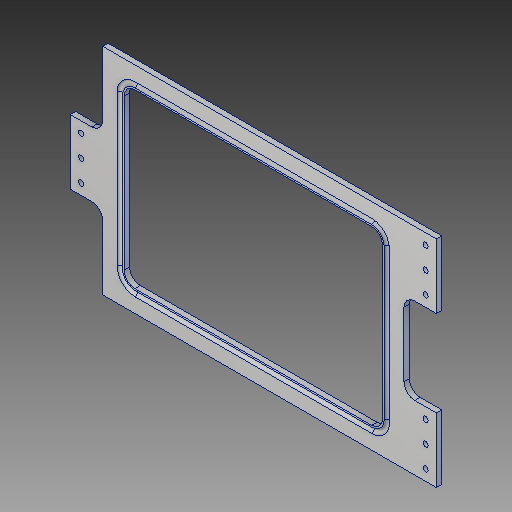
# Autodesk Inventor part: top
Saved by Autodesk Inventor 2018.1 (Build 221171000, 171)
## iProperties
Created: 2017-07-28
Part Number: top
Material: Aluminum 6061
Document SubType Name: Modeling
Designer: Kai
Density: 2.7 g/cm^3
Appearance: Aluminum - Flat
Author: Kai
Autodesk Inventor part; units mm, degrees
ref_plane "YZ Plane" through (0, 0, 0) normal (1, 0, 0) x (0, 1, 0)
ref_plane "XZ Plane" through (0, 0, 0) normal (0, 1, 0) x (-1, 0, 0)
sketch "Sketch1" plane through (0, 0, 0) normal (0, 0, 1) x (1, 0, 0)
  line L0 (0, 0) -> (-355.6, 0)
  line L1 (-355.6, 0) -> (-355.6, 254)
  line L2 (-355.6, 254) -> (0, 254)
  line L3 (0, 254) -> (0, 0)
  line L4 (-38.1, 25.4) -> (-317.5, 25.4)
  line L5 (-330.2, 38.1) -> (-330.2, 215.9)
  line L6 (-317.5, 228.6) -> (-38.1, 228.6)
  line L7 (-25.4, 215.9) -> (-25.4, 38.1)
  line L8 (-12.7, 241.3) -> (-342.9, 241.3) construction
  line L9 (-342.9, 241.3) -> (-342.9, 12.7) construction
  line L10 (-342.9, 12.7) -> (-12.7, 12.7) construction
  line L11 (-12.7, 12.7) -> (-12.7, 241.3) construction
  circle A0 centre (-342.9, 241.3) radius 3.1
  circle A1 centre (-342.9, 215.9) radius 3.1
  circle A2 centre (-342.9, 190.5) radius 3.1
  circle A3 centre (-342.9, 165.1) radius 3.1
  circle A4 centre (-342.9, 139.7) radius 3.1
  circle A5 centre (-342.9, 114.3) radius 3.1
  circle A6 centre (-342.9, 88.9) radius 3.1
  circle A7 centre (-342.9, 63.5) radius 3.1
  circle A8 centre (-342.9, 38.1) radius 3.1
  circle A9 centre (-342.9, 12.7) radius 3.1
  circle A10 centre (-317.5, 241.3) radius 3.1
  circle A11 centre (-292.1, 241.3) radius 3.1
  circle A12 centre (-266.7, 241.3) radius 3.1
  circle A13 centre (-241.3, 241.3) radius 3.1
  circle A14 centre (-215.9, 241.3) radius 3.1
  circle A15 centre (-190.5, 241.3) radius 3.1
  circle A16 centre (-165.1, 241.3) radius 3.1
  circle A17 centre (-139.7, 241.3) radius 3.1
  circle A18 centre (-114.3, 241.3) radius 3.1
  circle A19 centre (-88.9, 241.3) radius 3.1
  circle A20 centre (-63.5, 241.3) radius 3.1
  circle A21 centre (-38.1, 241.3) radius 3.1
  circle A22 centre (-12.7, 241.3) radius 3.1
  circle A23 centre (-12.7, 215.9) radius 3.1
  circle A24 centre (-12.7, 190.5) radius 3.1
  circle A25 centre (-12.7, 165.1) radius 3.1
  circle A26 centre (-12.7, 139.7) radius 3.1
  circle A27 centre (-12.7, 114.3) radius 3.1
  circle A28 centre (-12.7, 88.9) radius 3.1
  circle A29 centre (-12.7, 63.5) radius 3.1
  circle A30 centre (-12.7, 38.1) radius 3.1
  circle A31 centre (-12.7, 12.7) radius 3.1
  circle A32 centre (-38.1, 12.7) radius 3.1
  circle A33 centre (-63.5, 12.7) radius 3.1
  circle A34 centre (-88.9, 12.7) radius 3.1
  circle A35 centre (-114.3, 12.7) radius 3.1
  circle A36 centre (-139.7, 12.7) radius 3.1
  circle A37 centre (-165.1, 12.7) radius 3.1
  circle A38 centre (-190.5, 12.7) radius 3.1
  circle A39 centre (-215.9, 12.7) radius 3.1
  circle A40 centre (-241.3, 12.7) radius 3.1
  circle A41 centre (-266.7, 12.7) radius 3.1
  circle A42 centre (-292.1, 12.7) radius 3.1
  circle A43 centre (-317.5, 12.7) radius 3.1
  arc A44 (-317.5, 228.6) -> (-330.2, 215.9) centre (-317.5, 215.9) ccw
  arc A45 (-330.2, 38.1) -> (-317.5, 25.4) centre (-317.5, 38.1) ccw
  arc A46 (-38.1, 25.4) -> (-25.4, 38.1) centre (-38.1, 38.1) ccw
  arc A47 (-25.4, 215.9) -> (-38.1, 228.6) centre (-38.1, 215.9) ccw
  dimension "d0" = 355.6
  dimension "d1" = 254
  dimension "d2" = 25.4
  dimension "d3" = 12.7
  dimension "d4" = 6.2
  dimension "d7" = 25.4
  dimension "d14" = 25.4
  dimension "d21" = 25.4
  dimension "d28" = 25.4
  dimension "d33" = 12.7
  constraints: 48 centre point, 24 end point, 8 point on circle, 8 tangent, 6 parallel, 3 equal radius, 3 horizontal, 3 perpendicular, 2 vertical, 1 coincident, 92 other
  measures "d0" distance of L1.end L2.end
  measures "d1" distance of L0.end L1.end
  measures "d2" distance between parallel lines of L3 L7
  measures "d3" distance between parallel lines of L2 L8
  measures "d4" diameter of A0
  measures "d7" distance of A0.centre A1.centre
  measures "d14" distance of A0.centre A10.centre
  measures "d21" distance of A22.centre A23.centre
  measures "d28" distance of A31.centre A32.centre
  measures "d33" radius of A44
extrude "Extrusion1" add sketch "Sketch1" along normal blind 6.35
sketch "Sketch5" plane through (0, 0, 6.35) normal (0, 0, 1) x (1, 0, 0)
  arc A0 (-38.1, 25.4) -> (-25.4, 38.1) centre (-38.1, 38.1) ccw construction
  circle A1 centre (-12.7, 38.1) radius 3.1 construction
  circle A2 centre (-38.1, 38.1) radius 25.4 construction
  arc A3 (-330.2, 38.1) -> (-317.5, 25.4) centre (-317.5, 38.1) ccw construction
  circle A4 centre (-317.5, 38.1) radius 25.4 construction
  circle A5 centre (-342.9, 215.9) radius 3.1 construction
  circle A6 centre (-317.5, 215.9) radius 25.4 construction
  circle A7 centre (-12.7, 215.9) radius 3.1 construction
  circle A8 centre (-38.1, 215.9) radius 25.4 construction
  line L0 (-38.1, 215.9) -> (-20.1395, 233.8605) construction
  line L1 (-38.1, 215.9) -> (-12.7, 215.9) construction
  line L2 (-38.1, 38.1) -> (-20.1395, 20.1395) construction
  line L3 (-317.5, 38.1) -> (-335.4605, 20.1395) construction
  line L4 (-317.5, 215.9) -> (-335.4605, 233.8605) construction
  circle A9 centre (-335.4605, 233.8605) radius 3.1
  circle A10 centre (-20.1395, 233.8605) radius 3.1
  circle A11 centre (-20.1395, 20.1395) radius 3.1
  circle A12 centre (-335.4605, 20.1395) radius 3.1
  point P0 (0, 0)
  dimension "d49" = 45
  dimension "d50" = 6.2
  dimension "d51" = 6.2
  dimension "d52" = 6.2
  dimension "d53" = 6.2
  constraints: 10 end point, 7 centre point, 6 coincident, 6 point on circle, 2 perpendicular, 1 equal length, 1 horizontal, 3 other
  measures "d49" angle of L1 L0
  measures "d50" diameter of A9
  measures "d51" diameter of A10
  measures "d52" diameter of A11
  measures "d53" diameter of A12
extrude "Extrusion3" cut sketch "Sketch5" against normal blind 6.35
sketch "Sketch9" plane through (0, 0, 6.35) normal (0, 0, 1) x (1, 0, 0)
  circle A0 centre (-20.1395, 20.1395) radius 3.1 projected
  circle A1 centre (-20.1395, 20.1395) radius 3.1
  circle A2 centre (-38.1, 12.7) radius 3.1 projected
  circle A3 centre (-38.1, 12.7) radius 3.1
  circle A4 centre (-335.4605, 20.1395) radius 3.1 projected
  circle A5 centre (-335.4605, 20.1395) radius 3.1
  circle A6 centre (-335.4605, 233.8605) radius 3.1 projected
  circle A7 centre (-335.4605, 233.8605) radius 3.1
  circle A8 centre (-20.1395, 233.8605) radius 3.1 projected
  circle A9 centre (-20.1395, 233.8605) radius 3.1
  circle A10 centre (-38.1, 241.3) radius 3.1 projected
  circle A11 centre (-38.1, 241.3) radius 3.1
  circle A12 centre (-266.7, 241.3) radius 3.1 projected
  line L0 (-266.7, 241.3) -> (-275.1476, 241.3) construction
  line L1 (-292.1, 241.3) -> (-300.5476, 241.3) construction
  circle A13 centre (-63.5, 241.3) radius 3.1
  line L2 (-317.5, 241.3) -> (-325.9476, 241.3) construction
  circle A14 centre (-88.9, 241.3) radius 3.1
  line L3 (-342.9, 241.3) -> (-351.3476, 241.3) construction
  circle A15 centre (-114.3, 241.3) radius 3.1
  line L4 (-368.3, 241.3) -> (-376.7476, 241.3) construction
  circle A16 centre (-139.7, 241.3) radius 3.1
  line L5 (-393.7, 241.3) -> (-402.1476, 241.3) construction
  circle A17 centre (-165.1, 241.3) radius 3.1
  line L6 (-419.1, 241.3) -> (-427.5476, 241.3) construction
  circle A18 centre (-190.5, 241.3) radius 3.1
  line L7 (-444.5, 241.3) -> (-452.9476, 241.3) construction
  circle A19 centre (-215.9, 241.3) radius 3.1
  line L8 (-469.9, 241.3) -> (-478.3476, 241.3) construction
  circle A20 centre (-241.3, 241.3) radius 3.1
  line L9 (-495.3, 241.3) -> (-503.7476, 241.3) construction
  circle A21 centre (-266.7, 241.3) radius 3.1
  line L10 (-520.7, 241.3) -> (-529.1476, 241.3) construction
  circle A22 centre (-292.1, 241.3) radius 3.1
  line L11 (-546.1, 241.3) -> (-554.5476, 241.3) construction
  circle A23 centre (-317.5, 241.3) radius 3.1
  circle A24 centre (-342.9, 215.9) radius 3.1 projected
  circle A25 centre (-342.9, 215.9) radius 3.1
  line L12 (-342.9, 190.5569) -> (-342.9, 174.56) construction
  circle A26 centre (-63.5, 12.7) radius 3.1 construction
  line L13 (-63.5, 12.7) -> (-88.9, 12.7) construction
  circle A27 centre (-12.7, 38.1) radius 3.1 construction
  circle A28 centre (-12.7, 63.5) radius 3.1 construction
  line L14 (-12.7, 38.1) -> (-12.7, 63.5) construction
  circle A29 centre (-12.7, 215.9) radius 3.1 projected
  circle A30 centre (-12.7, 215.9) radius 3.1
  circle A31 centre (-12.7, 190.5) radius 3.1
  circle A32 centre (-12.7, 165.1) radius 3.1
  circle A33 centre (-12.7, 139.7) radius 3.1
  circle A34 centre (-12.7, 114.3) radius 3.1
  circle A35 centre (-12.7, 88.9) radius 3.1
  circle A36 centre (-12.7, 63.5) radius 3.1
  circle A37 centre (-12.7, 38.1) radius 3.1
  circle A38 centre (-63.5, 12.7) radius 3.1
  circle A39 centre (-88.9, 12.7) radius 3.1
  circle A40 centre (-114.3, 12.7) radius 3.1
  circle A41 centre (-139.7, 12.7) radius 3.1
  circle A42 centre (-165.1, 12.7) radius 3.1
  circle A43 centre (-190.5, 12.7) radius 3.1
  circle A44 centre (-215.9, 12.7) radius 3.1
  circle A45 centre (-241.3, 12.7) radius 3.1
  circle A46 centre (-266.7, 12.7) radius 3.1
  circle A47 centre (-292.1, 12.7) radius 3.1
  circle A48 centre (-317.5, 12.7) radius 3.1
  circle A49 centre (-342.9, 190.5) radius 3.1
  circle A50 centre (-342.9, 165.1) radius 3.1
  circle A51 centre (-342.9, 139.7) radius 3.1
  circle A52 centre (-342.9, 114.3) radius 3.1
  circle A53 centre (-342.9, 88.9) radius 3.1
  circle A54 centre (-342.9, 63.5) radius 3.1
  circle A55 centre (-342.9, 38.1) radius 3.1
  line L15 (-355.6, 254) -> (0, 254) projected
  line L16 (-355.6, 254) -> (0, 254)
  line L17 (0, 254) -> (0, 0)
  line L18 (0, 0) -> (-355.6, 0)
  line L19 (-355.6, 0) -> (-355.6, 254)
  dimension "d66" = 25.4
  dimension "d73" = 25.4
  dimension "d80" = 25.4
  dimension "d87" = 25.4
  constraints: 44 centre point, 38 end point, 8 coincident, 5 horizontal, 4 vertical, 2 parallel, 1 collinear, 1 perpendicular, 104 other
  measures "d66" distance of L0.start L1.start
  measures "d73" distance of A30.centre A31.centre
  measures "d80" distance of A3.centre A38.centre
  measures "d87" distance of A25.centre A49.centre
extrude "Extrusion4" add sketch "Sketch9" against normal blind 12.7
sketch "Sketch10" plane through (0, 0, 6.35) normal (0, 0, 1) x (1, 0, 0)
  line L0 (-355.6, 0) -> (-355.6, 254) construction
  line L1 (0, 0) -> (-355.6, 0) construction
  line L2 (-355.6, 0) -> (-355.6, 254) construction
  line L3 (-355.6, 254) -> (0, 254) construction
  line L4 (0, 254) -> (0, 0) construction
  line L5 (-38.1, 228.6) -> (-317.5, 228.6)
  line L6 (-330.2, 215.9) -> (-330.2, 38.1)
  line L7 (-317.5, 25.4) -> (-38.1, 25.4)
  line L8 (-25.4, 38.1) -> (-25.4, 215.9)
  arc A0 (-317.5, 228.6) -> (-330.2, 215.9) centre (-317.5, 215.9) ccw
  arc A1 (-25.4, 215.9) -> (-38.1, 228.6) centre (-38.1, 215.9) ccw
  arc A2 (-38.1, 25.4) -> (-25.4, 38.1) centre (-38.1, 38.1) ccw
  arc A3 (-330.2, 38.1) -> (-317.5, 25.4) centre (-317.5, 38.1) ccw
  dimension "d94" = 25.4
  dimension "d95" = 12.7
  constraints: 16 end point, 8 point on circle, 8 tangent, 4 centre point, 4 parallel, 3 equal radius, 2 perpendicular, 1 horizontal, 3 other
  measures "d94" distance between parallel lines of L3 L5
  measures "d95" radius of A0
extrude "Extrusion5" cut sketch "Sketch10" against normal blind 25.4
sketch "Sketch11" plane through (0, 0, -6.35) normal (0, 0, -1) x (-1, 0, 0)
  line L0 (355.6, 0) -> (355.6, 254) projected
  line L1 (0, 0) -> (355.6, 0)
  line L2 (355.6, 0) -> (355.6, 254)
  line L3 (355.6, 254) -> (0, 254)
  line L4 (0, 254) -> (0, 0)
  constraints: 8 end point, 2 parallel, 1 horizontal, 1 perpendicular
extrude "Extrusion6" cut sketch "Sketch11" against normal blind 6.35
sketch "Sketch12" plane through (0, 0, 6.35) normal (0, 0, 1) x (1, 0, 0)
  line L0 (-38.1, 20.32) -> (-317.5, 20.32)
  line L1 (-335.28, 38.1) -> (-335.28, 215.9)
  line L2 (-317.5, 233.68) -> (-38.1, 233.68)
  line L3 (-20.32, 215.9) -> (-20.32, 38.1)
  line L4 (-355.6, 254) -> (-355.6, 0) projected
  line L5 (-355.6, 0) -> (0, 0) projected
  arc A0 (-335.28, 38.1) -> (-317.5, 20.32) centre (-317.5, 38.1) ccw
  arc A1 (-317.5, 233.68) -> (-335.28, 215.9) centre (-317.5, 215.9) ccw
  arc A2 (-20.32, 215.9) -> (-38.1, 233.68) centre (-38.1, 215.9) ccw
  arc A3 (-38.1, 20.32) -> (-20.32, 38.1) centre (-38.1, 38.1) ccw
  point P0 (-335.28, 233.68)
  point P1 (-335.28, 20.32)
  point P2 (-20.32, 233.68)
  dimension "d100" = 314.96
  dimension "d101" = 213.36
  dimension "d102" = 20.32
  dimension "d103" = 20.32
  dimension "d104" = 17.78
  constraints: 8 end point, 8 point on circle, 8 tangent, 6 point on line, 4 centre point, 3 equal radius, 2 parallel, 1 horizontal, 1 perpendicular
  measures "d100" distance of point (-335.28, 233.68) point (-20.32, 233.68)
  measures "d101" distance of point (-335.28, 20.32) point (-335.28, 233.68)
  measures "d102" distance between parallel lines of L4 L1
  measures "d103" distance between parallel lines of L5 L0
  measures "d104" radius of A0
ref_plane "Work Plane2" through (-279.4, 38.1, 6.35) normal (1, 0, 0) x (0, 0, -1)
sketch "Sketch13" plane through (-279.4, 38.1, 6.35) normal (1, 0, 0) x (0, 0, -1)
  line L0 (0, 215.9) -> (0, -38.1) projected
  circle A0 centre (0, -17.78) radius 3.175
  line L1 (0, -38.1) -> (6.35, -38.1) projected
  dimension "d106" = 6.35
  dimension "d107" = 20.32
  constraints: 1 centre point, 1 point on line
  measures "d106" diameter of A0
  measures "d107" distance from line of L1 A0.centre
sweep "Sweep3" cut profiles "Sketch13" path "Sketch12" path curves L0 A3 L3 A2 L2 A1 L1 A0
sketch "Sketch14" plane through (0, 0, 6.35) normal (0, 0, 1) x (1, 0, 0)
  circle A0 centre (-20.1395, 20.1395) radius 3.1 projected
  circle A1 centre (-20.1395, 20.1395) radius 3.1
  circle A2 centre (-38.1, 12.7) radius 3.1 projected
  circle A3 centre (-38.1, 12.7) radius 3.1
  circle A4 centre (-12.7, 38.1) radius 3.1 projected
  circle A5 centre (-12.7, 38.1) radius 3.1
  circle A6 centre (-20.1395, 233.8605) radius 3.1 projected
  circle A7 centre (-20.1395, 233.8605) radius 3.1
  circle A8 centre (-38.1, 241.3) radius 3.1 projected
  circle A9 centre (-38.1, 241.3) radius 3.1
  circle A10 centre (-335.4605, 233.8605) radius 3.1 projected
  circle A11 centre (-335.4605, 233.8605) radius 3.1
  circle A12 centre (-335.4605, 20.1395) radius 3.1 projected
  circle A13 centre (-335.4605, 20.1395) radius 3.1
  circle A14 centre (-342.9, 38.1) radius 3.1 projected
  circle A15 centre (-342.9, 38.1) radius 3.1
  circle A16 centre (-292.1, 12.7) radius 3.1 construction
  circle A17 centre (-266.7, 12.7) radius 3.1 construction
  line L0 (-292.1, 12.7) -> (-266.7, 12.7) construction
  circle A18 centre (-342.9, 63.5) radius 3.1 construction
  circle A19 centre (-342.9, 88.9) radius 3.1 construction
  line L1 (-342.9, 63.5) -> (-342.9, 88.9) construction
  circle A20 centre (-292.1, 241.3) radius 3.1 construction
  line L2 (-292.1, 241.3) -> (-266.7, 241.3) construction
  circle A21 centre (-12.7, 215.9) radius 3.1 construction
  circle A22 centre (-12.7, 190.5) radius 3.1 construction
  line L3 (-12.7, 215.9) -> (-12.7, 190.5) construction
  circle A23 centre (-63.5, 241.3) radius 3.1
  circle A24 centre (-88.9, 241.3) radius 3.1
  circle A25 centre (-114.3, 241.3) radius 3.1
  circle A26 centre (-139.7, 241.3) radius 3.1
  circle A27 centre (-165.1, 241.3) radius 3.1
  circle A28 centre (-190.5, 241.3) radius 3.1
  circle A29 centre (-215.9, 241.3) radius 3.1
  circle A30 centre (-241.3, 241.3) radius 3.1
  circle A31 centre (-266.7, 241.3) radius 3.1
  circle A32 centre (-292.1, 241.3) radius 3.1
  circle A33 centre (-317.5, 241.3) radius 3.1
  circle A34 centre (-12.7, 63.5) radius 3.1
  circle A35 centre (-12.7, 88.9) radius 3.1
  circle A36 centre (-12.7, 114.3) radius 3.1
  circle A37 centre (-12.7, 139.7) radius 3.1
  circle A38 centre (-12.7, 165.1) radius 3.1
  circle A39 centre (-12.7, 190.5) radius 3.1
  circle A40 centre (-12.7, 215.9) radius 3.1
  circle A41 centre (-63.5, 12.7) radius 3.1
  circle A42 centre (-88.9, 12.7) radius 3.1
  circle A43 centre (-114.3, 12.7) radius 3.1
  circle A44 centre (-139.7, 12.7) radius 3.1
  circle A45 centre (-165.1, 12.7) radius 3.1
  circle A46 centre (-190.5, 12.7) radius 3.1
  circle A47 centre (-215.9, 12.7) radius 3.1
  circle A48 centre (-241.3, 12.7) radius 3.1
  circle A49 centre (-266.7, 12.7) radius 3.1
  circle A50 centre (-292.1, 12.7) radius 3.1
  circle A51 centre (-317.5, 12.7) radius 3.1
  circle A52 centre (-342.9, 63.5) radius 3.1
  circle A53 centre (-342.9, 88.9) radius 3.1
  circle A54 centre (-342.9, 114.3) radius 3.1
  circle A55 centre (-342.9, 139.7) radius 3.1
  circle A56 centre (-342.9, 165.1) radius 3.1
  circle A57 centre (-342.9, 190.5) radius 3.1
  circle A58 centre (-342.9, 215.9) radius 3.1
  point P0 (0, 0)
  dimension "d112" = 25.4
  dimension "d119" = 25.4
  dimension "d126" = 25.4
  dimension "d133" = 25.4
  constraints: 44 centre point, 8 coincident, 8 end point, 4 horizontal, 4 vertical, 72 other
  measures "d112" distance of A9.centre A23.centre
  measures "d119" distance of A5.centre A34.centre
  measures "d126" distance of A3.centre A41.centre
  measures "d133" distance of A15.centre A52.centre
extrude "Extrusion7" add sketch "Sketch14" against normal blind 6.35
sketch "Sketch15" plane through (0, 0, 6.35) normal (0, 0, 1) x (1, 0, 0)
  line L0 (-355.6, 254) -> (-355.6, 0) projected
  line L1 (-355.6, 165.1) -> (-393.7, 165.1)
  line L2 (-393.7, 165.1) -> (-393.7, 88.9)
  line L3 (-393.7, 88.9) -> (-355.6, 88.9)
  line L4 (-355.6, 88.9) -> (-355.6, 165.1)
  line L5 (0, 254) -> (-355.6, 254) projected
  line L6 (0, 254) -> (38.1, 254)
  line L7 (38.1, 254) -> (38.1, 177.8)
  line L8 (38.1, 177.8) -> (0, 177.8)
  line L9 (0, 177.8) -> (0, 254)
  line L10 (-355.6, 0) -> (0, 0) projected
  line L11 (0, 0) -> (38.1, 0)
  line L12 (38.1, 0) -> (38.1, 76.2)
  line L13 (38.1, 76.2) -> (0, 76.2)
  line L14 (0, 76.2) -> (0, 0)
  line L15 (-381, 165.1) -> (-381, 88.9) construction
  line L16 (25.4, 254) -> (25.4, 0) construction
  circle A0 centre (-381, 152.4) radius 3.1
  circle A1 centre (-381, 127) radius 3.1
  circle A2 centre (-381, 101.6) radius 3.1
  circle A3 centre (25.4, 241.3) radius 3.1
  circle A4 centre (25.4, 215.9) radius 3.1
  circle A5 centre (25.4, 190.5) radius 3.1
  circle A6 centre (25.4, 63.5) radius 3.1
  circle A7 centre (25.4, 38.1) radius 3.1
  circle A8 centre (25.4, 12.7) radius 3.1
  dimension "d140" = 38.1
  dimension "d141" = 76.2
  dimension "d142" = 88.9
  dimension "d143" = 38.1
  dimension "d144" = 76.2
  dimension "d145" = 38.1
  dimension "d146" = 76.2
  dimension "d147" = 12.7
  dimension "d148" = 12.7
  dimension "d149" = 6.2
  dimension "d150" = 12.7
  dimension "d153" = 25.4
  dimension "d158" = 6.2
  dimension "d159" = 12.7
  dimension "d162" = 25.4
  dimension "d167" = 6.2
  dimension "d168" = 12.7
  dimension "d171" = 25.4
  constraints: 28 end point, 9 centre point, 8 point on line, 6 parallel, 5 perpendicular, 3 horizontal, 3 vertical, 12 other
  measures "d140" distance of L3.end L2.end
  measures "d141" distance of L2.end L1.end
  measures "d142" distance between parallel lines of L5 L1
  measures "d143" distance of L7.end L8.end
  measures "d144" distance of L6.end L7.end
  measures "d145" distance of L13.end L12.end
  measures "d146" distance of L12.end L11.end
  measures "d147" distance between parallel lines of L16 L12
  measures "d148" distance between parallel lines of L2 L15
  measures "d149" diameter of A0
  measures "d150" distance from line of L1 A0.centre
  measures "d153" distance of A0.centre A1.centre
  measures "d158" diameter of A3
  measures "d159" distance from line of A3.centre L6
  measures "d162" distance of A3.centre A4.centre
  measures "d167" diameter of A6
  measures "d168" distance from line of L13 A6.centre
  measures "d171" distance of A6.centre A7.centre
extrude "Extrusion8" add sketch "Sketch15" against normal blind 6.35
fillet "Fillet2" radius 12.7 4 edges at (-355.6, 88.9, 3.175) (-355.6, 165.1, 3.175) (0, 76.2, 3.175) (0, 177.8, 3.175)
body "Solid1"
